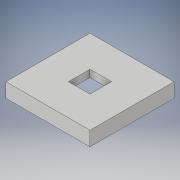
# Autodesk Inventor part: test_camera_seat
Saved by Autodesk Inventor 2018 (Build 220112000, 112)
## iProperties
Created: 2020-03-27
Part Number: test_camera_seat
Material: Generic
Document SubType Name: Modeling
Designer: natha
Density: 1 g/cm^3
Appearance: Default
Author: natha
Autodesk Inventor part; units mm, degrees
ref_plane "YZ Plane" through (0, 0, 0) normal (1, 0, 0) x (0, 1, 0)
ref_plane "XZ Plane" through (0, 0, 0) normal (0, 1, 0) x (-1, 0, 0)
ref_plane "XY Plane" through (0, 0, 0) normal (0, 0, 1) x (1, 0, 0)
sketch "Sketch1" plane through (0, 0, 0) normal (0, 1, 0) x (-1, 0, 0)
  line L0 (0.5335, -0.6929) -> (33.0335, -0.6929)
  line L1 (33.0335, -0.6929) -> (33.0335, -33.1929)
  line L2 (33.0335, -33.1929) -> (0.5335, -33.1929)
  line L3 (0.5335, -33.1929) -> (0.5335, -0.6929)
  line L4 (-0.7165, 0.5571) -> (34.2835, 0.5571)
  line L5 (34.2835, 0.5571) -> (34.2835, -34.4429)
  line L6 (34.2835, -34.4429) -> (-0.7165, -34.4429)
  line L7 (-0.7165, -34.4429) -> (-0.7165, 0.5571)
  point P0 (0, 0)
  dimension "d0" = 32.5
  dimension "d1" = 32.5
  dimension "d2" = 35
  dimension "d3" = 35
  dimension "d4" = 1.25
  dimension "d5" = 1.25
  constraints: 16 end point, 4 parallel, 2 horizontal, 2 perpendicular
  measures "d0" distance of L1.end L2.end
  measures "d1" distance of L0.end L1.end
  measures "d2" distance of L5.end L6.end
  measures "d3" distance of L4.end L5.end
  measures "d4" distance between parallel lines of L4 L0
  measures "d5" distance between parallel lines of L3 L7
extrude "Extrusion1" add sketch "Sketch1" along normal blind 3
sketch "Sketch2" plane through (0, 3, 0) normal (0, 1, 0) x (1, 0, 0)
  line L0 (-34.2835, -0.5571) -> (0.7165, -0.5571) projected
  line L1 (0.7165, -0.5571) -> (0.7165, 34.4429) projected
  line L2 (-34.2835, -0.5571) -> (0.7165, -0.5571)
  line L3 (0.7165, -0.5571) -> (0.7165, 34.4429)
  line L4 (0.7165, 34.4429) -> (-34.2835, 34.4429)
  line L5 (-34.2835, 34.4429) -> (-34.2835, -0.5571)
  point P0 (0, 0)
  constraints: 8 end point, 2 parallel, 1 horizontal, 1 perpendicular
extrude "Extrusion2" add sketch "Sketch2" along normal blind 3
sketch "Sketch3" plane through (0, 6, 0) normal (0, 1, 0) x (1, 0, 0)
  line L0 (-21.2835, 12.4429) -> (-12.2835, 12.4429)
  line L1 (-12.2835, 12.4429) -> (-12.2835, 21.4429)
  line L2 (-12.2835, 21.4429) -> (-21.2835, 21.4429)
  line L3 (-21.2835, 21.4429) -> (-21.2835, 12.4429)
  line L4 (-34.2835, 34.4429) -> (-34.2835, -0.5571) projected
  line L5 (0.7165, 34.4429) -> (-34.2835, 34.4429) projected
  point P0 (0, 0)
  dimension "d10" = 9
  dimension "d11" = 9
  dimension "d12" = 13
  dimension "d13" = 13
  constraints: 8 end point, 2 parallel, 1 horizontal, 1 perpendicular
  measures "d10" distance of L2.end L1.end
  measures "d11" distance of L1.end L0.end
  measures "d12" distance between parallel lines of L4 L3
  measures "d13" distance between parallel lines of L5 L2
extrude "Extrusion3" cut sketch "Sketch3" against normal blind 3
body "Solid1"
